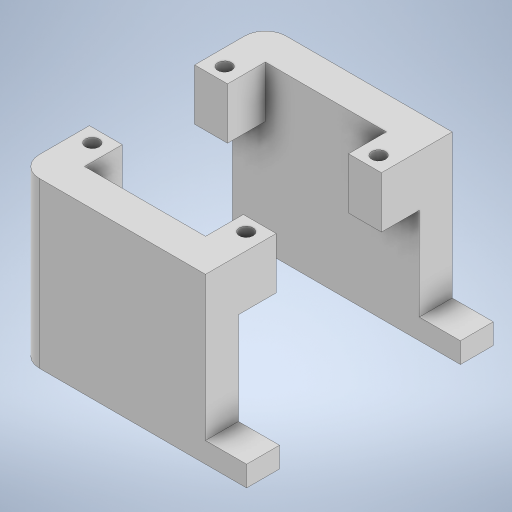
# Autodesk Inventor part: lepton mount
Saved by Autodesk Inventor 2024 (Build 280153000, 153)
## iProperties
Created: 2024-01-12
Part Number: lepton mount
Material: Generic
Document SubType Name: Modeling
Designer: Eli
Density: 1 g/cm^3
Appearance: Default
Author: Eli
Autodesk Inventor part; units mm, degrees
note: some values were not read from the file. Chosen so that the rebuilt part matches the saved one: direction of "Hole1".
ref_plane "YZ Plane" through (0, 0, 0) normal (1, 0, 0) x (0, 1, 0)
ref_plane "XZ Plane" through (0, 0, 0) normal (0, 1, 0) x (-1, 0, 0)
sketch "Sketch1" plane through (0, 0, 0) normal (0, 1, 0) x (-1, 0, 0)
  line L0 (0, 0) -> (-8.9535, 0)
  line L1 (-8.9535, 0) -> (-8.9535, -82.296)
  line L2 (-8.9535, -82.296) -> (0, -82.296)
  line L3 (0, -82.296) -> (0, 0)
  line L4 (0, -41.148) -> (-8.9535, -41.148) construction
  line L5 (0, -22.098) -> (19.9009, -22.098)
  line L6 (19.9009, -22.098) -> (19.9009, -60.198)
  line L7 (19.9009, -60.198) -> (0, -60.198)
  line L8 (0, -60.198) -> (0, -22.098)
  line L9 (19.9009, -55.118) -> (0, -55.118)
  line L10 (0, -55.118) -> (0, -27.178)
  line L11 (0, -27.178) -> (19.9009, -27.178)
  line L12 (19.9009, -27.178) -> (19.9009, -55.118)
  line L13 (0, -55.118) -> (8.9662, -55.118)
  line L14 (8.9662, -55.118) -> (8.9662, -27.178)
  line L15 (8.9662, -27.178) -> (0, -27.178)
  line L16 (0, -27.178) -> (0, -55.118)
  line L17 (0, -27.178) -> (-8.9535, -27.178)
  line L18 (0, -55.118) -> (-8.9535, -55.118)
  line L19 (0, -22.098) -> (-8.9535, -22.098)
  line L20 (0, -60.198) -> (-8.9535, -60.198)
  line L21 (-8.9535, -27.178) -> (-21.6535, -27.178)
  line L22 (-21.6535, -27.178) -> (-21.6535, -14.478)
  line L23 (-21.6535, -14.478) -> (-15.3035, -14.478)
  line L24 (-8.9535, -13.6415) -> (-8.9535, -27.178)
  line L25 (-8.9535, -55.118) -> (-16.891, -55.118)
  line L26 (-16.891, -67.818) -> (-8.9535, -67.818)
  line L27 (-8.9535, -67.818) -> (-8.9535, -55.118)
  line L28 (-8.9535, -22.098) -> (-15.3035, -22.098)
  line L29 (-15.3035, -22.098) -> (-15.3035, -14.478)
  line L30 (-15.3035, -22.098) -> (-15.3035, -27.178)
  point P0 (-4.4768, 0)
  point P1 (0, -60.198)
  point P2 (0, -55.118)
  point P3 (19.9009, -27.178)
  point P4 (0, -55.118)
  point P5 (0, -60.198)
  point P6 (-8.9535, -67.818)
  point P7 (-8.9535, -13.6415)
  dimension "d0" = 82.296
  dimension "d1" = 8.9535
  dimension "d5" = 38.1
  dimension "d6" = 19.9009
  dimension "d11" = 27.94
  dimension "d28" = 8.9662
  dimension "d46" = 7.9375
  dimension "d48" = 12.7
  dimension "d50" = 12.7
  dimension "d51" = 6.35
  dimension "d52" = 6.35
  constraints: 62 end point, 11 parallel, 9 perpendicular, 8 point on line, 7 horizontal, 4 midpoint, 2 other
  measures "d0" distance of L0.end L1.end
  measures "d1" distance of L0.start L0.end
  measures "d5" distance of L5.end L6.end
  measures "d6" distance between parallel lines of L8 L6
  measures "d11" distance between parallel lines of L11 L9
  measures "d28" distance between parallel lines of L8 L14
  measures "d46" distance of L26.start L26.end
  measures "d48" distance of L25.end L26.start
  measures "d50" distance of L21.end L22.end
  measures "d51" distance of L22.end L23.end
  measures "d52" distance between parallel lines of L1 L29
extrude "Extrusion1" add sketch "Sketch1" along normal blind 3.175 contours L1 L21 L30 L28
extrude "Extrusion2" add sketch "Sketch1" along normal blind 25.4 contours L5 L6 L11 L3 | L3 L17 L1 L19 | L9 L6 L7 L3 | L3 L20 L1 L18
sketch "Sketch2" plane through (-19.9009, 0, -55.118) normal (0, 0, 1) x (1, 0, 0)
  line L0 (23.7744, 25.4) -> (23.7744, 17.4625)
  line L1 (23.7744, 17.4625) -> (28.8544, 17.4625)
  line L2 (28.8544, 17.4625) -> (28.8544, 25.4)
  line L3 (28.8544, 0) -> (28.8544, 25.4) projected
  line L4 (23.7744, 25.4) -> (28.8544, 25.4)
  line L5 (28.8544, 25.4) -> (28.8544, 17.4625)
  line L6 (19.9009, 0) -> (19.9009, 0) projected
  line L7 (0, 25.4) -> (28.8544, 25.4) projected
  point P0 (28.8544, 3.175)
  point P1 (36.7919, 0)
  dimension "d40" = 7.9375
  dimension "d41" = 5.08
  dimension "d44" = 7.9375
  constraints: 10 end point, 1 parallel, 1 perpendicular, 1 other
  measures "d40" distance of L0.start L0.end
  measures "d41" distance of L0.end L1.end
  measures "d44" distance between parallel lines of L7 L1
extrude "Extrusion3" add sketch "Sketch2" along normal blind 5.842
sketch "Sketch3" plane through (0, 25.4, 0) normal (0, 1, 0) x (1, 0, 0)
  line L0 (-19.9009, 55.118) -> (8.9535, 55.118) construction
  line L1 (3.8735, 49.276) -> (8.9535, 49.276) construction
  line L2 (6.4135, 49.276) -> (6.4135, 55.118) construction
  line L3 (-19.9009, 55.118) -> (8.9535, 55.118) construction
  point P0 (0, 0)
  point P1 (0, 55.118)
  point P2 (6.4135, 51.3715)
  point P3 (-8.9662, 55.118)
  point P4 (16.891, 55.118)
  dimension "d34" = 2.0955
  dimension "d35" = 0
  constraints: 2 end point, 1 midpoint, 1 point on line, 1 vertical
  measures "d34" distance from line of L1 point (6.413, 51.371)
  measures "d35" distance from line of L2 point (6.413, 51.371)
hole "Hole1" at (6.4135, 25.4, -51.3715) direction (0, -1, 0) diameter 2.1463 depth 7.9375
ref_plane "Work Plane4" through (-19.9009, 0, -41.148) normal (0, 0, 1) x (1, 0, 0)
mirror "Mirror3" about plane through (-19.9009, 0, -41.148) normal (0, 0, 1) of "Hole1", "Extrusion3"
fillet "Fillet11" radius 3.175 2 edges at (-19.9009, 12.7, -22.098) (-19.9009, 12.7, -60.198)
ref_plane "Work Plane5" through (-5.4737, 3.175, -22.098) normal (1, 0, 0) x (0, 0, -1)
mirror "Mirror5" about plane through (-5.4737, 3.175, -22.098) normal (1, 0, 0) of "Hole1", "Extrusion3", "Mirror3"
mirror "Mirror6" about plane through (-19.9009, 0, -41.148) normal (0, 0, 1) of "Extrusion1"
body "Solid1"
